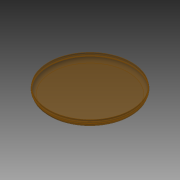
# Autodesk Inventor part: DisceepSL_CaseBottom
Saved by Autodesk Inventor 2014 (Build 180170000, 170)
## iProperties
Created: 2014-11-22
Part Number: DisceepSL_CaseBottom
Material: Polycarbonate, Smoke
Document SubType Name: Modeling
Designer: DV
Mass: 0.0164458 g
Surface Area: 5.41694 cm^2
Volume: 0.0137049 cm^3
Density: 1.2 g/cm^3
Appearance: Polycarbonate - Smoked
Author: DV
Autodesk Inventor part; units mm, degrees
ref_plane "YZ Plane" through (0, 0, 0) normal (1, 0, 0) x (0, 1, 0)
ref_plane "XZ Plane" through (0, 0, 0) normal (0, 1, 0) x (-1, 0, 0)
ref_plane "XY Plane" through (0, 0, 0) normal (0, 0, 1) x (1, 0, 0)
sketch "Sketch1" plane through (0, 0, 0) normal (0, 0, 1) x (1, 0, 0)
  line L0 (8.1006, -2.5834) -> (-8.1006, -2.5834) projected
  arc A0 (-8.1006, -2.5834) -> (-8.1493, -2.8276) centre (-8.1006, -2.7104) ccw
  line L1 (1.4612, -3.605) -> (-5.2946, -3.605) projected
  line L2 (0, -3.605) -> (-7.4732, -3.605)
  line L3 (-8.1082, -2.97) -> (-8.1082, -2.8893)
  arc A1 (-8.1082, -2.97) -> (-7.4732, -3.605) centre (-7.4732, -2.97) ccw
  arc A2 (-8.1082, -2.8893) -> (-8.1493, -2.8276) centre (-8.175, -2.8893) ccw
  line L4 (8.1006, -2.8374) -> (-6.8522, -2.8374)
  line L5 (-8.1006, -2.5834) -> (-8.1006, -2.2677)
  line L6 (0, -3.6558) -> (-7.4732, -3.6558)
  arc A3 (-8.159, -2.97) -> (-7.4732, -3.6558) centre (-7.4732, -2.97) ccw
  line L7 (-8.159, -2.97) -> (-8.159, -2.8893)
  arc A4 (-8.159, -2.8893) -> (-8.1688, -2.8746) centre (-8.175, -2.8893) ccw
  arc A5 (-8.1514, -2.54) -> (-8.1688, -2.8746) centre (-8.1006, -2.7104) ccw
  line L8 (-8.1514, -2.54) -> (-8.1514, -2.2677)
  arc A6 (-8.1006, -2.2677) -> (-8.1514, -2.2677) centre (-8.126, -2.2677) ccw
  line L9 (0, -3.6558) -> (0, -3.605)
  point P0 (0, 0)
  point P1 (-8.1082, -3.605)
  dimension "d0" = 0.635
  dimension "d1" = 0.0508
  constraints: 16 end point, 15 point on circle, 7 centre point, 6 tangent, 4 point on line, 1 horizontal, 1 parallel, 1 perpendicular, 6 other
  measures "d0" radius of A1
  measures "d1" distance between parallel lines of L6 L2
revolve "Revolution1" add sketch "Sketch1" angle 360 about axis through (0, -3.6558, 0) along (0, 1, 0)
body "Solid1"
